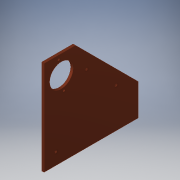
# Autodesk Inventor part: level 2
Saved by Autodesk Inventor 2017 (Build 210142000, 142)
## iProperties
Created: 2017-03-06
Part Number: level 2
Material: Copper
Document SubType Name: Modeling
Designer: vitor
Density: 8.94 g/cm^3
Appearance: Copper - Satin
Author: vitor
Autodesk Inventor part; units mm, degrees
ref_plane "YZ Plane" through (0, 0, 0) normal (1, 0, 0) x (0, 1, 0)
ref_plane "XZ Plane" through (0, 0, 0) normal (0, 1, 0) x (-1, 0, 0)
ref_plane "XY Plane" through (0, 0, 0) normal (0, 0, 1) x (1, 0, 0)
sketch "Sketch1" plane through (0, 0, 0) normal (1, 0, 0) x (0, 1, 0)
  line L0 (60, 60) -> (-60, 60)
  line L1 (-60, 60) -> (-60, -60)
  line L2 (60, 20) -> (60, 60)
  line L3 (60, 60) -> (60, 20)
  line L4 (60, 20) -> (-20, -60)
  line L5 (-20, -60) -> (-60, -60)
  point P0 (0, 0)
  point P1 (-60, 0)
  point P2 (0, 60)
  dimension "d1" = 120
  dimension "d2" = 40
  dimension "d3" = 40
  dimension "d5" = 90
  constraints: 12 end point, 2 horizontal, 2 midpoint, 1 horizontal alignment, 1 parallel, 1 vertical alignment
  measures "d1" distance of L1.end L0.end
  measures "d2" distance of L1.end L4.end
  measures "d3" distance of L2.start L0.start
  measures "d5" angle of L0 L1
extrude "Extrusion1" add sketch "Sketch1" along normal blind 3
sketch "Sketch2" plane through (3, 0, 0) normal (1, 0, 0) x (0, 0, -1)
  circle A0 centre (-38, 36) radius 15
  line L0 (-20, 60) -> (-60, 60) projected
  line L1 (-60, 60) -> (-60, -60) projected
  line L2 (60, -60) -> (60, -20) projected
  line L3 (-60, -60) -> (60, -60) projected
  line L4 (60, -20) -> (-20, 60) projected
  circle A1 centre (31.7157, -10) radius 10
  circle A2 centre (-45, -45) radius 10
  circle A3 centre (-6, 26.5414) radius 10
  circle A4 centre (-45, -45) radius 1.5
  circle A5 centre (31.7157, -10) radius 1.5
  circle A6 centre (-6, 26.5414) radius 1.5
  circle A7 centre (-34.7007, 17.2887) radius 1.25
  circle A8 centre (-41.2993, 54.7113) radius 1.25
  line L5 (-38, 36) -> (-41.2993, 54.7113) construction
  line L6 (-38, 36) -> (-19, 36) construction
  line L7 (-38, 36) -> (-34.7007, 17.2887) construction
  line L8 (-38, 36) -> (-19, 36) construction
  point P0 (0, 0)
  dimension "d8" = 30
  dimension "d9" = 24
  dimension "d10" = 22
  dimension "d69" = 20
  dimension "d70" = 20
  dimension "d71" = 30
  dimension "d72" = 50
  dimension "d73" = 15
  dimension "d74" = 15
  dimension "d75" = 20
  dimension "d76" = 54
  dimension "d77" = 3
  dimension "d78" = 3
  dimension "d79" = 3
  dimension "d84" = 2.5
  dimension "d85" = 2.5
  dimension "d88" = 19
  dimension "d89" = 100
  dimension "d90" = 19
  dimension "d91" = 80
  constraints: 9 centre point, 8 end point, 5 coincident, 2 equal length, 2 horizontal
  measures "d8" diameter of A0
  measures "d9" distance from line of L5.start L0
  measures "d10" distance from line of L5.start L1
  measures "d69" diameter of A1
  measures "d70" diameter of A2
  measures "d71" distance of L2.end A1.centre
  measures "d72" distance from line of L3 A1.centre
  measures "d73" distance from line of L1 A2.centre
  measures "d74" distance from line of L3 A2.centre
  measures "d75" diameter of A3
  measures "d76" distance from line of L1 A3.centre
  measures "d77" diameter of A4
  measures "d78" diameter of A5
  measures "d79" diameter of A6
  measures "d84" diameter of A7
  measures "d85" diameter of A8
  measures "d88" distance of L5.start L5.end
  measures "d89" angle of L6 L5
  measures "d90" distance of L5.start L7.end
  measures "d91" angle of L7 L8
extrude "Extrusion3" cut sketch "Sketch2" against normal blind 3 contours A0 | A4 | A5 | A6 | A7 | A8
body "Solid1"
